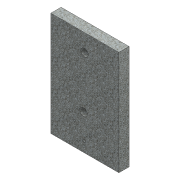
# Autodesk Inventor part: protoPlinth
Saved by Autodesk Inventor 2017 (Build 210142000, 142)
## iProperties
Created: 2017-05-18
Part Number: protoPlinth
Material: Generic
Document SubType Name: Modeling
Designer: krosie
Density: 1 g/cm^3
Appearance: Exposed Aggregate - Warm Gray
Author: krosie
Autodesk Inventor part; units mm, degrees
ref_plane "YZ Plane" through (0, 0, 0) normal (1, 0, 0) x (0, 1, 0)
ref_plane "XZ Plane" through (0, 0, 0) normal (0, 1, 0) x (-1, 0, 0)
ref_plane "XY Plane" through (0, 0, 0) normal (0, 0, 1) x (1, 0, 0)
sketch "Sketch1" plane through (0, 0, 0) normal (0, 1, 0) x (-1, 0, 0)
  circle A0 centre (0, 0) radius 55
  line L0 (480, 1020) -> (-520, 1020)
  line L1 (-520, 1020) -> (-520, -515)
  line L2 (-520, -515) -> (480, -515)
  line L3 (480, -515) -> (480, 1020)
  line L4 (267, -266) -> (-327, -266) construction
  circle A1 centre (132, -175) radius 15
  circle A2 centre (-97, -255) radius 15
  circle A3 centre (-8, -360) radius 20
  circle A4 centre (-15, 765) radius 55
  dimension "d0" = 110
  dimension "d1" = 515
  dimension "d2" = 1020
  dimension "d3" = 520
  dimension "d4" = 480
  dimension "d5" = 30
  dimension "d6" = 30
  dimension "d7" = 40
  dimension "d8" = 155
  dimension "d9" = 255
  dimension "d10" = 340
  dimension "d11" = 110
  dimension "d13" = 505
  dimension "d14" = 765
  constraints: 10 end point, 5 centre point, 2 horizontal, 2 parallel, 1 coincident, 1 perpendicular
  measures "d0" diameter of A0
  measures "d1" distance from line of L2 point (0, 0)
  measures "d2" distance from line of L0 point (0, 0)
  measures "d3" distance from line of L1 point (0, 0)
  measures "d4" distance from line of L3 point (0, 0)
  measures "d5" diameter of A1
  measures "d6" diameter of A2
  measures "d7" diameter of A3
  measures "d8" distance from line of L2 A3.centre
  measures "d9" vertical distance of A2.centre point (0, 0)
  measures "d10" distance from line of L2 A1.centre
  measures "d11" diameter of A4
  measures "d13" distance from line of L1 A4.centre
  measures "d14" vertical distance of point (0, 0) A4.centre
extrude "Extrusion1" add sketch "Sketch1" along normal blind 150
body "Solid1"
